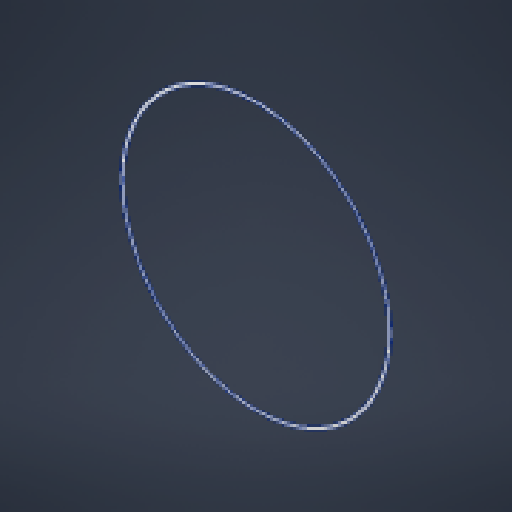
# Autodesk Inventor part: Former
Saved by Autodesk Inventor 2026.2 (Build 302298000, 298)
## iProperties
Created: 2026-02-13
Part Number: Former
Material: Aluminum 6061
Document SubType Name: Modeling
Designer: Lex Machina
Density: 2.7 g/cm^3
Appearance: Aluminum - Flat
Mass: 7108.17 g
Surface Area: 14216.3 cm^2
Volume: 2632.65 cm^3
Author: Lex Machina
Autodesk Inventor part; units mm, degrees
ref_plane "YZ Plane" through (0, 0, 0) normal (1, 0, 0) x (0, 1, 0)
ref_plane "XZ Plane" through (0, 0, 0) normal (0, 1, 0) x (-1, 0, 0)
ref_plane "XY Plane" through (0, 0, 0) normal (0, 0, 1) x (1, 0, 0)
sketch "Sketch1" plane through (0, 0, 0) normal (0, 0, 1) x (1, 0, 0)
  circle A0 centre (0, 0) radius 2120
  dimension "d0" = 4240
  constraints: 1 centre point, 1 coincident
  measures "d0" diameter of A0
extrude "Extrusion1" add sketch "Sketch1" along normal blind 4
shell "Shell1" thickness 50 removed faces 2 at (720.9234, 751.8276, 4) at (720.9234, 751.8276, 0)
body "Solid1"
